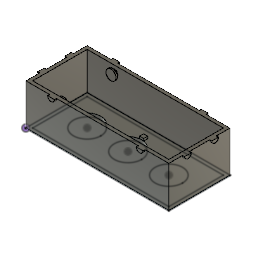
case top v4 (Autodesk Fusion 360 design; units mm, degrees)
Autodesk Fusion 360 part; units mm, degrees
note: some values were not read from the file. Set by a fixed rule: which sketch regions a step uses.
sketch "Sketch1" plane through (0, 0, 0) normal (0, 0, 1) x (1, 0, 0)
  line L0 (0, 0) -> (210, 0)
  line L1 (210, 0) -> (210, 90)
  line L2 (210, 90) -> (0, 90)
  line L3 (0, 90) -> (0, 0)
  line L4 (5, 5) -> (205, 5)
  line L5 (205, 5) -> (205, 85)
  line L6 (205, 85) -> (5, 85)
  line L7 (5, 85) -> (5, 5)
  circle A0 centre (45, 45) radius 20
  circle A1 centre (105, 45) radius 20
  circle A2 centre (165, 45) radius 20
  dimension "d1" = 210
  dimension "d2" = 90
  dimension "d3" = 200
  dimension "d4" = 80
  dimension "d5" = 5
  dimension "d6" = 5
  dimension "d7" = 40
  dimension "d8" = 40
  dimension "d9" = 40
  dimension "d10" = 105
  dimension "d11" = 45
  dimension "d12" = 45
  dimension "d13" = 45
  dimension "d14" = 60
  dimension "d15" = 60
  constraint horizontal L0
  constraint vertical L1
  constraint horizontal L2
  constraint vertical L3
  constraint coincident L0.start L3.end
  constraint horizontal L4
  constraint vertical L5
  constraint horizontal L6
  constraint vertical L7
  measures "d1" distance of L0.start L0.end
  measures "d2" distance of L0.start L2.end
  measures "d3" distance of L4.start L4.end
  measures "d4" distance of L4.start L6.end
  measures "d5" distance of L0 L4
  measures "d6" distance of L3 L7
  measures "d7" diameter of A0
  measures "d8" diameter of A1
  measures "d9" diameter of A2
  measures "d10" distance of L1 A1.centre
  measures "d11" distance of L0 A1.centre
  measures "d12" distance of L0 A2.centre
  measures "d13" distance of L0 A0.centre
  measures "d14" distance of A1.centre A2.centre
  measures "d15" distance of A0.centre A1.centre
extrude "Extrude1" add sketch "Sketch1" along normal blind 5 contours L4 L5 L6 L7
extrude "Extrude2" add sketch "Sketch1" along normal blind 60 contours L0 L1 L2 L3
sketch "Sketch2" plane through (210, 0, 0) normal (1, 0, 0) x (0, 1, 0)
  line L0 (0, 0) -> (90, 0)
  line L1 (90, 0) -> (90, 60)
  line L2 (90, 60) -> (0, 60)
  line L3 (0, 60) -> (0, 0)
  circle A0 centre (25, 60) radius 5
  circle A1 centre (65, 60) radius 5
  line L4 (20, 60) -> (30, 60)
  line L5 (60, 60) -> (70, 60)
  dimension "d20" = 10
  dimension "d21" = 10
  dimension "d22" = 25
  dimension "d23" = 25
  constraint coincident L2 A0.centre
  constraint coincident L2 A1.centre
  constraint coincident A0 L4.start
  constraint coincident L2 L4.start
  constraint coincident A0 L4.end
  constraint coincident L2 L4.end
  constraint coincident A1 L5.start
  constraint coincident L2 L5.start
  constraint coincident A1 L5.end
  constraint coincident L2 L5.end
  measures "d20" diameter of A1
  measures "d21" diameter of A0
  measures "d22" distance of L1 A1.centre
  measures "d23" distance of L2.end A0.centre
extrude "Extrude3" add sketch "Sketch2" along normal blind 3 contours L2 A0 L4 | L2 A1 L5 picked at (25.8333, 56.3489) picked at (63.59, 57.0721)
sketch "Sketch3" plane through (0, 0, 0) normal (0, -1, 0) x (1, 0, 0)
  line L0 (0, 0) -> (210, 0)
  line L1 (210, 0) -> (210, 60)
  line L2 (210, 60) -> (0, 60)
  line L3 (0, 60) -> (0, 0)
  circle A0 centre (40, 60) radius 5
  circle A1 centre (170, 60) radius 5
  line L4 (35, 60) -> (45, 60)
  line L5 (165, 60) -> (175, 60)
  dimension "d26" = 10
  dimension "d27" = 10
  dimension "d28" = 40
  dimension "d29" = 40
  constraint coincident L2 A0.centre
  constraint coincident L2 A1.centre
  constraint coincident A0 L4.start
  constraint coincident L2 L4.start
  constraint coincident A0 L4.end
  constraint coincident L2 L4.end
  constraint coincident A1 L5.start
  constraint coincident L2 L5.start
  constraint coincident A1 L5.end
  constraint coincident L2 L5.end
  measures "d26" diameter of A0
  measures "d27" diameter of A1
  measures "d28" distance of L1 A1.centre
  measures "d29" distance of L2.end A0.centre
extrude "Extrude4" add sketch "Sketch3" along normal blind 3 contours L2 A0 L4 | L2 A1 L5 picked at (38.8698, 57.4825) picked at (169.3911, 57.9517)
ref_plane "WorkPlane1" through (105, 45, 30) normal (0, -1, 0) x (1, 0, 0)
ref_plane "WorkPlane2" through (105, 0, 0) normal (1, 0, 0) x (0, 1, 0)
mirror "Mirror1" about plane through (105, 45, 30) normal (0, -1, 0) of bodies 1 merged
mirror "Mirror2" about plane through (105, 0, 0) normal (1, 0, 0) of bodies 1 merged
sketch "Sketch4" plane through (0, 85, 0) normal (0, -1, 0) x (1, 0, 0)
  line L0 (5, 5) -> (205, 5)
  line L1 (205, 5) -> (205, 60)
  line L2 (205, 60) -> (5, 60)
  line L3 (5, 60) -> (5, 5)
  circle A0 centre (45, 50) radius 5
  line L4 (0, 0) -> (0, 60)
  dimension "d38" = 45
  dimension "d39" = 10
  measures "d38" distance of A0.centre L4
  measures "d39" distance of L2 A0.centre
extrude "Extrude5" add sketch "Sketch4" along normal blind 5 contours A0
sketch "Sketch5" plane through (0, 80, 0) normal (0, -1, 0) x (1, 0, 0)
  circle A0 centre (45, 50) radius 5
  circle A1 centre (45, 50) radius 7.5
  dimension "d42" = 15
  constraint concentric A0 A1
  measures "d42" diameter of A1
extrude "Extrude6" add sketch "Sketch5" against normal blind 2
mirror "Mirror3" about plane through (105, 45, 30) normal (0, -1, 0) of bodies 1 merged
sketch "Sketch6" plane through (0, 0, 5) normal (0, 0, 1) x (-1, 0, 0)
  arc A0 (-65, -45) -> (-25, -45) centre (-45, -45) ccw
  arc A1 (-25, -45) -> (-65, -45) centre (-45, -45) ccw
  arc A2 (-125, -45) -> (-85, -45) centre (-105, -45) ccw
  arc A3 (-85, -45) -> (-125, -45) centre (-105, -45) ccw
  arc A4 (-185, -45) -> (-145, -45) centre (-165, -45) ccw
  arc A5 (-145, -45) -> (-185, -45) centre (-165, -45) ccw
  line L0 (-5, -85) -> (-5, -5)
  line L1 (-5, -5) -> (-205, -5)
  line L2 (-205, -5) -> (-205, -85)
  line L3 (-205, -85) -> (-5, -85)
  line L4 (-102, -71) -> (-108, -71)
  line L5 (-108, -71) -> (-108, -65)
  line L6 (-108, -65) -> (-102, -65)
  line L7 (-102, -65) -> (-102, -71)
  line L8 (-102, -25) -> (-108, -25)
  line L9 (-108, -25) -> (-108, -19)
  line L10 (-108, -19) -> (-102, -19)
  line L11 (-102, -19) -> (-102, -25)
  circle A6 centre (-105, -45) radius 20
  line L12 (-210, 0) -> (-210, -90)
  line L13 (-102, -71) -> (-108, -71)
  line L14 (-108, -71) -> (-108, -73)
  line L15 (-108, -73) -> (-102, -73)
  line L16 (-102, -73) -> (-102, -71)
  line L17 (-108, -69) -> (-110, -69)
  line L18 (-110, -69) -> (-110, -67)
  line L19 (-110, -67) -> (-108, -67)
  line L20 (-108, -67) -> (-108, -69)
  line L21 (-102, -69) -> (-100, -69)
  line L22 (-100, -69) -> (-100, -67)
  line L23 (-100, -67) -> (-102, -67)
  line L24 (-102, -67) -> (-102, -69)
  line L25 (-108, -19) -> (-102, -19)
  line L26 (-102, -19) -> (-102, -17)
  line L27 (-102, -17) -> (-108, -17)
  line L28 (-108, -17) -> (-108, -19)
  line L29 (-108, -23) -> (-110, -23)
  line L30 (-110, -23) -> (-110, -21)
  line L31 (-110, -21) -> (-108, -21)
  line L32 (-108, -21) -> (-108, -23)
  line L33 (-102, -23) -> (-100, -23)
  line L34 (-100, -23) -> (-100, -21)
  line L35 (-100, -21) -> (-102, -21)
  line L36 (-102, -21) -> (-102, -23)
  dimension "d47" = 6
  dimension "d48" = 6
  dimension "d49" = 6
  dimension "d50" = 6
  dimension "d51" = 102
  dimension "d52" = 2
  dimension "d53" = 2
  dimension "d54" = 2
  dimension "d55" = 2
  dimension "d56" = 2
  dimension "d57" = 2
  dimension "d58" = 2
  dimension "d63" = 6
  dimension "d64" = 2
  dimension "d65" = 2
  dimension "d66" = 2
  dimension "d67" = 2
  dimension "d68" = 2
  dimension "d69" = 2
  dimension "d70" = 2
  constraint horizontal L4
  constraint vertical L5
  constraint horizontal L6
  constraint vertical L7
  constraint horizontal L8
  constraint vertical L9
  constraint horizontal L10
  constraint vertical L11
  constraint tangent L6 A6
  constraint tangent L8 A6
  constraint collinear L5 L9
  constraint horizontal L13
  constraint vertical L14
  constraint horizontal L15
  constraint vertical L16
  constraint horizontal L17
  constraint vertical L18
  constraint horizontal L19
  constraint vertical L20
  constraint coincident L5 L17.start
  constraint horizontal L21
  constraint vertical L22
  constraint horizontal L23
  constraint vertical L24
  constraint coincident L7 L21.start
  constraint collinear L5 L14
  constraint horizontal L25
  constraint vertical L26
  constraint horizontal L27
  constraint vertical L28
  constraint horizontal L29
  constraint vertical L30
  constraint horizontal L31
  constraint vertical L32
  constraint coincident L9 L29.start
  constraint horizontal L33
  constraint vertical L34
  constraint horizontal L35
  constraint vertical L36
  constraint coincident L11 L33.start
  measures "d47" distance of L4.start L4.end
  measures "d48" distance of L4.start L6.end
  measures "d49" distance of L8.start L8.end
  measures "d50" distance of L8.start L10.end
  measures "d51" distance of L4.end L12
  measures "d52" distance of L4.start L15.end
  measures "d53" distance of L17.start L17.end
  measures "d54" distance of L17.start L19.end
  measures "d55" distance of L21.start L23.end
  measures "d56" distance of L22.end L23.end
  measures "d57" distance of L13 L17
  measures "d58" distance of L4 L21
  measures "d63" distance of L9.end L10.end
  measures "d64" distance of L9.end L27.end
  measures "d65" distance of L29.start L29.end
  measures "d66" distance of L29.start L31.end
  measures "d67" distance of L33.start L33.end
  measures "d68" distance of L33.start L35.end
  measures "d69" distance of L9.end L31
  measures "d70" distance of L10 L35
extrude "Extrude7" add sketch "Sketch6" along normal blind 3 contours L4 L5 L6 L7 L13 L20 L24
extrude "Extrude8" add sketch "Sketch6" along normal blind 2 contours L11 L33 L34 L35 L36 | L9 L29 L30 L31 L32 | L10 L25 L26 L27 L28
